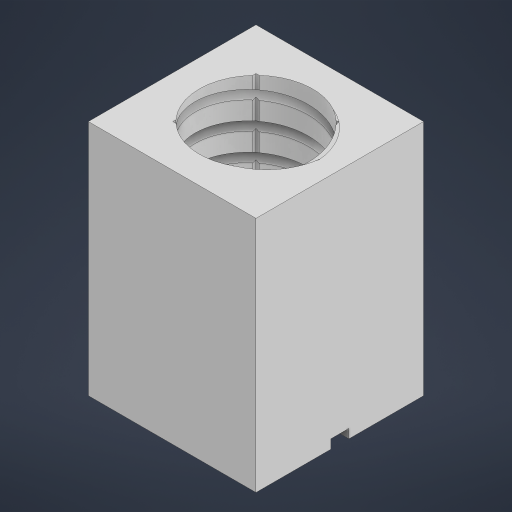
# Autodesk Inventor part: Oxy_A
Saved by Autodesk Inventor 2024.1 (Build 281209000, 209)
## iProperties
Created: 2024-08-16
Part Number: Oxy_A
Material: Generic
Document SubType Name: Modeling
Designer: Tim Jäger
Density: 1 g/cm^3
Appearance: Default
Author: Tim Jäger
## iProperties of the stored document Oxy_A_3DPrint.ipt
Created: 2024-08-17
Part Number: Oxy_A_3DPrint
Material: Generic
Document SubType Name: Modeling
Designer: Tim Jäger
Density: 1 g/cm^3
Appearance: Default
Author: Tim Jäger
Autodesk Inventor part; units mm, degrees
ref_plane "YZ Plane" through (0, 0, 0) normal (1, 0, 0) x (0, 1, 0)
ref_plane "XZ Plane" through (0, 0, 0) normal (0, 1, 0) x (-1, 0, 0)
ref_plane "XY Plane" through (0, 0, 0) normal (0, 0, 1) x (1, 0, 0)
sketch "Sketch1" plane through (0, 0, 0) normal (0, 1, 0) x (-1, 0, 0)
  line L0 (-7.5, 7.5) -> (7.5, 7.5)
  line L1 (7.5, 7.5) -> (7.5, -7.5)
  line L2 (7.5, -7.5) -> (-7.5, -7.5)
  line L3 (-7.5, -7.5) -> (-7.5, 7.5)
  line L4 (-7.5, 7.5) -> (7.5, -7.5) construction
  line L5 (7.5, 7.5) -> (-7.5, -7.5) construction
  line L6 (-18.5, -18.5) -> (18.5, -18.5)
  line L7 (18.5, -18.5) -> (18.5, 18.5)
  line L8 (18.5, 18.5) -> (-18.5, 18.5)
  line L9 (-18.5, 18.5) -> (-18.5, -18.5)
  point P0 (0, 0)
  dimension "d0" = 15
  dimension "d1" = 15
  dimension "d2" = 37
  constraints: 20 end point, 4 parallel, 2 midpoint, 2 perpendicular, 1 horizontal, 3 other
  measures "d0" distance of L1.end L2.end
  measures "d1" distance of L0.end L1.end
  measures "d2" distance of L6.start L6.end
extrude "Extrusion1" add sketch "Sketch1" along normal blind 2
sketch "Sketch2" plane through (0, 2, 0) normal (0, 1, 0) x (1, 0, 0)
  line L0 (-18.5, 18.5) -> (-18.5, -18.5) projected
  line L1 (-18.5, -18.5) -> (18.5, -18.5) projected
  line L2 (18.5, -18.5) -> (18.5, 18.5) projected
  line L3 (18.5, 18.5) -> (-18.5, 18.5) projected
  line L4 (7.5, -7.5) -> (-7.5, -7.5) construction
  line L5 (-7.5, -7.5) -> (-7.5, 7.5) construction
  line L6 (-7.5, 7.5) -> (7.5, 7.5) construction
  line L7 (7.5, 7.5) -> (7.5, -7.5) construction
  line L8 (9.18, 9.18) -> (-9.18, 9.18)
  line L9 (-9.18, 9.18) -> (-9.18, -9.18)
  line L10 (-9.18, -9.18) -> (9.18, -9.18)
  line L11 (9.18, -9.18) -> (9.18, 9.18)
  line L12 (9.18, 9.18) -> (-9.18, -9.18) construction
  line L13 (-9.18, 9.18) -> (9.18, -9.18) construction
  point P0 (0, 0)
  dimension "d6" = 18.36
  dimension "d7" = 18.36
  constraints: 12 end point, 2 midpoint, 2 parallel, 1 horizontal, 1 perpendicular
  measures "d6" distance of L10.end L9.end
  measures "d7" distance of L9.end L8.end
extrude "Extrusion2" add sketch "Sketch2" along normal blind 0.4
sketch "Sketch3" plane through (0, 2.4, 0) normal (0, 1, 0) x (1, 0, 0)
  circle A0 centre (0, 0) radius 12.5
  line L0 (-18.5, -18.5) -> (18.5, -18.5) projected
  line L1 (18.5, -18.5) -> (18.5, 18.5) projected
  line L2 (18.5, 18.5) -> (-18.5, 18.5) projected
  line L3 (-18.5, 18.5) -> (-18.5, -18.5) projected
  line L4 (9.18, 9.18) -> (9.18, -9.18) projected
  line L5 (9.18, -9.18) -> (-9.18, -9.18) projected
  line L6 (-9.18, -9.18) -> (-9.18, 9.18) projected
  line L7 (-9.18, 9.18) -> (9.18, 9.18) projected
  point P0 (8.484, 9.18)
  point P1 (9.18, 8.484)
  point P2 (9.18, -8.484)
  point P3 (8.484, -9.18)
  point P4 (-8.484, -9.18)
  point P5 (-9.18, -8.484)
  point P6 (-9.18, 8.484)
  point P7 (-8.484, 9.18)
  dimension "d10" = 25
  constraints: 1 centre point, 1 coincident
  measures "d10" diameter of A0
extrude "Extrusion3" add sketch "Sketch3" along normal blind 50
sketch "Sketch4" plane through (0, 0, 0) normal (1, 0, 0) x (0, 1, 0)
  line L0 (52.4, -12.5) -> (2.4, -12.5) projected
  line L1 (4.9, -12.5) -> (5.9, -14.2321)
  line L2 (5.9, -14.2321) -> (6.9, -12.5)
  point P0 (0, 0)
  dimension "d13" = 60
  dimension "d14" = 2.5
  dimension "d15" = 2
  constraints: 4 end point, 2 point on line, 1 equal length
  measures "d13" angle of L2 L1
  measures "d14" distance of L0.end L1.start
  measures "d15" distance of L2.end L1.start
coil "Coil1" sketch "Sketch4" operation cut axis through (0, -10, 0) along (0, 1, 0) pitch 6 turns 10 hand right
sketch "Sketch5" plane through (0, 2.4, 0) normal (0, 1, 0) x (1, 0, 0)
  circle A0 centre (0, 0) radius 12.5
  circle A1 centre (0, 0) radius 10.5
  arc A2 (-9.18, 8.484) -> (-9.18, -8.484) centre (0, 0) ccw projected
  line L0 (-9.18, -8.484) -> (-9.18, 8.484) projected
  arc A3 (-8.484, -9.18) -> (8.484, -9.18) centre (0, 0) ccw projected
  line L1 (8.484, -9.18) -> (-8.484, -9.18) projected
  arc A4 (8.484, 9.18) -> (-8.484, 9.18) centre (0, 0) ccw projected
  line L2 (-8.484, 9.18) -> (8.484, 9.18) projected
  arc A5 (9.18, -8.484) -> (9.18, 8.484) centre (0, 0) ccw projected
  line L3 (9.18, 8.484) -> (9.18, -8.484) projected
  point P0 (9.18, -5.0968)
  point P1 (9.18, -8.484)
  point P2 (9.18, 8.484)
  point P3 (9.18, 5.0968)
  point P4 (-5.0968, -9.18)
  point P5 (8.484, -9.18)
  point P6 (5.0968, -9.18)
  point P7 (-9.18, 5.0968)
  point P8 (-9.18, -8.484)
  point P9 (-9.18, -5.0968)
  point P10 (5.0968, 9.18)
  point P11 (-5.0968, 9.18)
  dimension "d24" = 21
  constraints: 2 coincident, 1 centre point, 3 other
  measures "d24" diameter of A1
extrude "Extrusion4" add sketch "Sketch5" along normal up to surface (2.5 mm away) contours A0 L3 A1 | L2 A1 A0 | A0 L1 A1 | L0 A1 A0
sketch "Sketch6" plane through (0, 0, 0) normal (0, -1, 0) x (1, 0, 0)
  line L0 (7.5, -7.5) -> (7.5, 7.5) projected
  line L1 (18.5, 18.5) -> (18.5, -18.5) projected
  line L2 (7.5, 2) -> (18.5, 2)
  line L3 (18.5, 2) -> (18.5, -2)
  line L4 (18.5, -2) -> (7.5, -2)
  line L5 (7.5, -2) -> (7.5, 2)
  point P0 (0, 0)
  point P1 (7.5, 0)
  point P2 (7.5, 0)
  dimension "d27" = 4
  constraints: 8 end point, 2 horizontal alignment, 2 midpoint, 2 parallel, 2 point on line, 1 horizontal, 1 perpendicular
  measures "d27" distance between parallel lines of L4 L2
extrude "Extrusion5" cut sketch "Sketch6" against normal up to surface (2 mm away)
body "Solid1"
